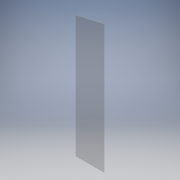
# Autodesk Inventor part: Side Walls
Saved by Autodesk Inventor 2017 (Build 210142000, 142)
## iProperties
Created: 2017-01-16
Part Number: Side Walls
Material: Polycarbonate, Clear
Document SubType Name: Modeling
Designer: Ben
Density: 1.2 g/cm^3
Appearance: Polycarbonate - Clear
Mass: 65.9067 g
Surface Area: 707.861 cm^2
Volume: 54.9223 cm^3
Author: Ben
Autodesk Inventor part; units mm, degrees
ref_plane "YZ Plane" through (0, 0, 0) normal (1, 0, 0) x (0, 1, 0)
ref_plane "XZ Plane" through (0, 0, 0) normal (0, 1, 0) x (-1, 0, 0)
ref_plane "XY Plane" through (0, 0, 0) normal (0, 0, 1) x (1, 0, 0)
sketch "Sketch1" plane through (0, 0, 0) normal (0, 0, 1) x (1, 0, 0)
  line L0 (0, 0) -> (82.55, 0)
  line L1 (82.55, 0) -> (82.55, 381)
  line L2 (82.55, 381) -> (0, 381)
  line L3 (0, 381) -> (0, 0)
  line L4 (73.025, 381) -> (73.025, 0) construction
  line L5 (82.55, 190.5) -> (0, 190.5) construction
  circle A0 centre (73.025, 190.5) radius 1.5875
  circle A1 centre (73.025, 107.95) radius 1.5875
  circle A2 centre (73.025, 25.4) radius 1.5875
  circle A3 centre (73.025, 273.05) radius 1.5875
  circle A4 centre (73.025, 355.6) radius 1.5875
  dimension "d0" = 82.55
  dimension "d1" = 381
  dimension "d7" = 9.525
  dimension "d16" = 3.175
  dimension "d19" = 82.55
  dimension "d26" = 82.55
  constraints: 12 end point, 5 centre point, 3 midpoint, 3 point on line, 2 parallel, 2 perpendicular, 2 vertical, 1 horizontal, 8 other
  measures "d0" distance of L0.start L0.end
  measures "d1" distance of L2.end L0.start
  measures "d7" distance of L0.end L4.end
  measures "d16" diameter of A0
  measures "d19" distance of A0.centre A1.centre
  measures "d26" distance of A0.centre A3.centre
extrude "Extrusion1" add sketch "Sketch1" along normal blind 1.5875
chamfer "Chamfer1" distance 82.55 angle 13 1 edges at (0, 381, 0.7937) measured on face at (55.0333, 381, 0.5292)
body "Solid1"
